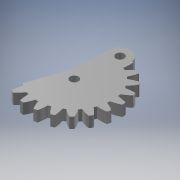
# Autodesk Inventor part: 平歯車2
Saved by Autodesk Inventor 2018 (Build 220112000, 112)
## iProperties
Created: 2017-10-29
Part Number: 平歯車2
Material: Steel
Document SubType Name: Modeling
Designer: sktom
Categories: <?xml version="1.0" encoding="UTF-16"?> <MemberInstance><Categories><FamilyTemplate><FamilyTemplateParameter ValueType="xs:double" Id="1" ObjectReferenceKey="da_z" ObjectType="kUserParameterObject"/><FamilyTemplateParameter ValueType="xs:double" Id="2" ObjectReferenceKey="da_b" ObjectType="kUserParameterObject"/><FamilyTemplateParameter ValueType="xs:double" Id="3" ObjectReferenceKey="da_beta" ObjectType="kUserParameterObject"/><FamilyTemplateParameter ValueType="xs:double" Id="4" ObjectReferenceKey="da_da" ObjectType="kUserParameterObject"/><FamilyTemplateParameter ValueType="xs:double" Id="5" ObjectReferenceKey="da_aw" ObjectType="kUserParameterObject"/><FamilyTemplateParameter ValueType="xs:string" Id="6" ObjectReferenceKey="EAIAABAAAACIAQAAAAAAAIAAAAAAAAAA" ObjectType="83910656" SubObjectId="SurfaceGeometry"/></FamilyTemplate><ParamToTemplateMap><ParamToTemplate CategoryParameter="//CategoryParameter[@InternalName='046C89C9-8512-4d59-83FE-43B91F4F132A']" TemplateParameter="1"/><ParamToTemplate CategoryParameter="//CategoryParameter[@InternalName='2552DF32-E462-4b46-AEBF-C6C7768E72AC']" TemplateParameter="2"/><ParamToTemplate CategoryParameter="//CategoryParameter[@InternalName='C9EE641D-15FC-4fae-A226-E94C4372FDD7']" TemplateParameter="3"/><ParamToTemplate><ParamToTemplate CategoryParameter="//CategoryParameter[@InternalName='00B6519A-459B-49c7-AD84-2E56D39A5744']" ConstantValue="0.000000"/></ParamToTemplate><ParamToTemplate><ParamToTemplate CategoryParameter="//CategoryParameter[@InternalName='04B31F0E-C7A6-4894-AA32-9629BEFACF47']" ConstantValue="1.000000"/></ParamToTemplate><ParamToTemplate><ParamToTemplate CategoryParameter="//CategoryParameter[@InternalName='43CBEC2E-7847-49e7-A936-2F7889FCB2D9']" ConstantValue="0.250000"/></ParamToTemplate><ParamToTemplate><ParamToTemplate CategoryParameter="//CategoryParameter[@InternalName='B1EFC894-105D-4ebd-86BF-FA20ED196853']" ConstantValue="0.350000"/></ParamToTemplate><ParamToTemplate><ParamToTemplate CategoryParameter="//CategoryParameter[@InternalName='51175063-3D10-4879-93E8-6246FE8B403D']" ConstantValue="2060000000.000000"/></ParamToTemplate><ParamToTemplate><ParamToTemplate CategoryParameter="//CategoryParameter[@InternalName='A3A52E27-4454-46a9-B0BD-C932399B70AF']" ConstantValue="0.300000"/></ParamToTemplate><ParamToTemplate><ParamToTemplate CategoryParameter="//CategoryParameter[@InternalName='91B76062-C214-41d9-B1B9-14D2AB99603D']" ConstantValue="0.100000"/></ParamToTemplate><ParamToTemplate><ParamToTemplate CategoryParameter="//CategoryParameter[@InternalName='374E806E-8B8A-4dda-A9AA-1039D6500AD2']" ConstantValue="10.000000"/></ParamToTemplate><ParamToTemplate><ParamToTemplate CategoryParameter="//CategoryParameter[@InternalName='2D373A89-B862-43d6-8D0B-0CBF12AB9F6C']" ConstantValue="0.349066"/></ParamToTemplate><ParamToTemplate CategoryParameter="//CategoryParameter[@InternalName='37777632-D6A2-4fac-9D53-DB8ACD95C989']" TemplateParameter="4"/><ParamToTemplate CategoryParameter="//CategoryParameter[@InternalName='FD1017F1-B727-4f7e-9707-0F86F1FF9423']" TemplateParameter="5"/><ParamToTemplate><ParamToTemplate CategoryParameter="//CategoryParameter[@InternalName='9E1B4470-B2D3-4ff1-B813-535BB4CDF51A']" ConstantValue="3520000.000000"/></ParamToTemplate><ParamToTemplate><ParamToTemplate CategoryParameter="//CategoryParameter[@InternalName='F8452263-BFF6-458c-9FB1-07C4B99E95CD']" ConstantValue="11400000.000000"/></ParamToTemplate><ParamToTemplate><ParamToTemplate CategoryParameter="//CategoryParameter[@InternalName='3E3BB259-FD49-497f-8171-6EBC954A3479']" ConstantValue="2.000000"/></ParamToTemplate><ParamToTemplate CategoryParameter="//CategoryParameter[@InternalName='27C3BAF2-7550-4e4b-AE2C-0DB134B7D9B7']" TemplateParameter="6"/></ParamToTemplateMap><Category DisplayName="Gear" InternalName="DC85795E-93AB-48d5-8EEE-5A27447B64BD" Mnemonic="Gear"><CategoryParameter DisplayName="z" InternalName="046C89C9-8512-4d59-83FE-43B91F4F132A" Mnemonic="z"/><CategoryParameter DisplayName="b" InternalName="2552DF32-E462-4b46-AEBF-C6C7768E72AC" Mnemonic="b"/><CategoryParameter DisplayName="||b|" InternalName="C9EE641D-15FC-4fae-A226-E94C4372FDD7" Mnemonic="beta"/><CategoryParameter DisplayName="x" InternalName="00B6519A-459B-49c7-AD84-2E56D39A5744" Mnemonic="x"/><CategoryParameter DisplayName="a*" InternalName="04B31F0E-C7A6-4894-AA32-9629BEFACF47" Mnemonic="a"/><CategoryParameter DisplayName="c*" InternalName="43CBEC2E-7847-49e7-A936-2F7889FCB2D9" Mnemonic="c"/><CategoryParameter DisplayName="r|.f|*" InternalName="B1EFC894-105D-4ebd-86BF-FA20ED196853" Mnemonic="rf"/><CategoryParameter DisplayName="E" InternalName="51175063-3D10-4879-93E8-6246FE8B403D" Mnemonic="E"/><CategoryParameter DisplayName="||m|" InternalName="A3A52E27-4454-46a9-B0BD-C932399B70AF" Mnemonic="mi"/><Category DisplayName="SpurGear" InternalName="26C5A22E-A91E-4dfd-A3B3-23CCAFAE1764" Mnemonic="SpurGear"><CategoryParameter DisplayName="m" InternalName="91B76062-C214-41d9-B1B9-14D2AB99603D" Mnemonic="m"/><CategoryParameter DisplayName="P" InternalName="374E806E-8B8A-4dda-A9AA-1039D6500AD2" Mnemonic="PP"/><CategoryParameter DisplayName="||a|" InternalName="2D373A89-B862-43d6-8D0B-0CBF12AB9F6C" Mnemonic="alpha"/><CategoryParameter DisplayName="d|.a|" InternalName="37777632-D6A2-4fac-9D53-DB8ACD95C989" Mnemonic="da"/><CategoryParameter DisplayName="a|.w|" InternalName="FD1017F1-B727-4f7e-9707-0F86F1FF9423" Mnemonic="aw"/><CategoryParameter DisplayName="||s||.Flim|" InternalName="9E1B4470-B2D3-4ff1-B813-535BB4CDF51A" Mnemonic="sFlim"/><CategoryParameter DisplayName="||s||.Hlim|" InternalName="F8452263-BFF6-458c-9FB1-07C4B99E95CD" Mnemonic="sHlim"/><CategoryParameter DisplayName="種類" InternalName="3E3BB259-FD49-497f-8171-6EBC954A3479" Mnemonic="type"/><CategoryParameter DisplayName="PitchDiameter" InternalName="27C3BAF2-7550-4e4b-AE2C-0DB134B7D9B7" Mnemonic="IDS_PITCHDIAM"/></Category></Category></Categories></MemberInstance>
Density: 1 g/cm^3
Appearance: Steel
CustomPartVersion: 1
Author: sktom
Autodesk Inventor part; units mm, degrees
ref_plane "YZ Plane" through (0, 0, 0) normal (1, 0, 0) x (0, 1, 0)
ref_plane "XZ Plane" through (0, 0, 0) normal (0, 1, 0) x (-1, 0, 0)
ref_plane "XY Plane" through (0, 0, 0) normal (0, 0, 1) x (1, 0, 0)
sketch "Sketch1" plane through (0, 0, 0) normal (0, 0, 1) x (1, 0, 0)
  circle A0 centre (0, 0) radius 11.5
  dimension "d0" = 23
  constraints: 1 centre point
  measures "d0" diameter of A0
extrude "Extrusion1" add sketch "Sketch1" along normal blind 2.651
ref_plane "Work Plane2" through (0, 0, 1.3255) normal (0, 0, 1) x (1, 0, 0)
sketch "Sketch2" plane through (0, 0, 0) normal (0, 0, -1) x (-1, 0, 0)
  circle A0 centre (0, 0) radius 11.5 projected
  circle A1 centre (0, 0) radius 10.5
  dimension "d3" = 21
  constraints: 1 centre point, 1 coincident
  measures "d3" diameter of A1
surface extrude "ピッチ円直径" sketch "Sketch2" against normal through all shown no curves A1
ref_plane "Work Plane8" through (0, 0, 0) normal (0.9888308, 0.1490423, 0) x (0, 0, 1)
ref_plane "Work Plane9" through (0, 0, 0) normal (1, 0, 0) x (0, 1, 0)
spur gear teeth "平歯車" teeth 21 pitch diameter 21 tip diameter 23 root diameter 18.5 face width 3 start plane through (0, 0, 0) normal (0, 0, -1) x (-1, 0, 0)
sketch "スケッチ3" plane through (0, 0, 2.651) normal (0, 0, 1) x (1, 0, 0)
  circle A0 centre (0, 0) radius 1.05
  dimension "d49" = 2.1
  constraints: 1 centre point, 1 coincident
  measures "d49" diameter of A0
extrude "押し出し2" cut sketch "スケッチ3" against normal through all
sketch "スケッチ4" plane through (0, 0, 2.651) normal (0, 0, 1) x (1, 0, 0)
  circle A0 centre (0.7711, 10.5759) radius 1.05
  circle A1 centre (0.7711, 10.5759) radius 2.651
  line L0 (-1.8729, 10.7687) -> (-2.5842, 1.0131)
  line L1 (-2.5842, 1.0131) -> (-8.2774, -10.3528)
  arc A2 (0.9638, 13.2199) -> (-8.2774, -10.3528) centre (0, 0) ccw
  line L2 (0, 0) -> (-12.3406, 4.8379) construction
  line L3 (0.7711, 10.5759) -> (0, 0) construction
  arc A3 (3.7982, 10.8547) -> (2.9764, 11.1081) centre (0, 0) ccw construction
  point P0 (3.3897, 10.9891)
  dimension "d52" = 10.604
  dimension "d53" = 2.1
  dimension "d54" = 157.563
  dimension "d55" = 2.651
  constraints: 8 end point, 7 point on circle, 3 centre point, 2 coincident, 2 tangent, 1 parallel, 1 point on line
  measures "d52" distance of point (0, 0) A0.centre
  measures "d53" diameter of A0
  measures "d54" angle of L0 L1
  measures "d55" distance from line of point (0, 0) L0
extrude "押し出し3" cut sketch "スケッチ4" against normal through all contours A1 L0 L1 A2
extrude "押し出し4" add sketch "スケッチ4" against normal up to surface (2.651 mm away) contours A1
extrude "押し出し5" cut sketch "スケッチ4" against normal through all contours A0
sketch "スケッチ5" plane through (0, 0, 2.651) normal (0, 0, 1) x (1, 0, 0)
  circle A0 centre (0.7711, 10.5759) radius 2.651 projected
  line L0 (-1.9591, 9.586) -> (-2.5842, 1.0131) projected
  line L1 (-1.8729, 10.7687) -> (-2.5842, 1.0131) projected
  line L2 (0.7711, 10.5759) -> (0, 0) construction
  line L3 (0.5783, 7.9319) -> (-2.0657, 8.1247)
  constraints: 2 end point, 2 point on line, 1 perpendicular, 1 point on circle, 1 tangent
extrude "押し出し6" add sketch "スケッチ5" against normal up to surface (2.651 mm away) contours A0 L3 L0 L1
fillet "フィレット1" radius 0.5 1 edges at (-7.445, -8.6909, 1.3255)
sketch "スケッチ6" plane through (0, 0, 2.651) normal (0, 0, 1) x (1, 0, 0)
  line L0 (-6.6843, -7.1724) -> (-2.5842, 1.0131) projected
  line L1 (-2.5842, 1.0131) -> (-6.9082, -7.6194)
  line L2 (-6.9082, -7.6194) -> (-6.1476, -8.0004)
  arc A0 (-5.4928, -7.4425) -> (-4.9213, -7.8322) centre (0, 0) ccw projected
  line L3 (-6.1476, -8.0004) -> (-5.4928, -7.4425)
  line L4 (-5.4928, -7.4425) -> (-2.5842, 1.0131)
  arc A1 (-6.6843, -7.1724) -> (-5.9392, -7.7978) centre (-6.2373, -7.3963) ccw projected
  arc A2 (-6.6843, -7.1724) -> (-5.9392, -7.7978) centre (-6.2373, -7.3963) ccw construction
  arc A3 (-5.9392, -7.7978) -> (-5.4928, -7.4425) centre (-11.0042, -0.9749) ccw construction
  arc A4 (-5.4928, -7.4425) -> (-4.9213, -7.8322) centre (0, 0) ccw construction
  arc A5 (-4.9213, -7.8322) -> (-5.3736, -10.1673) centre (3.1128, -10.5997) ccw construction
  arc A6 (-5.3736, -10.1673) -> (-4.5988, -10.5405) centre (0, 0) ccw construction
  arc A7 (-4.5988, -10.5405) -> (-3.0551, -8.7309) centre (-10.2279, -4.1751) ccw construction
  arc A8 (-3.0551, -8.7309) -> (-2.3941, -8.9348) centre (0, 0) ccw construction
  arc A9 (-2.3941, -8.9348) -> (-2.138, -11.2995) centre (6.0988, -9.2113) ccw construction
  arc A10 (-2.138, -11.2995) -> (-1.2876, -11.4277) centre (0, 0) ccw construction
  arc A11 (-1.2876, -11.4277) -> (-0.3459, -9.2435) centre (-8.5429, -7.0044) ccw construction
  arc A12 (-0.3459, -9.2435) -> (0.3459, -9.2435) centre (0, 0) ccw construction
  arc A13 (0.3459, -9.2435) -> (1.2876, -11.4277) centre (8.5429, -7.0044) ccw construction
  arc A14 (1.2876, -11.4277) -> (2.138, -11.2995) centre (0, 0) ccw construction
  arc A15 (2.138, -11.2995) -> (2.3941, -8.9348) centre (-6.0988, -9.2113) ccw construction
  arc A16 (2.3941, -8.9348) -> (3.0551, -8.7309) centre (0, 0) ccw construction
  arc A17 (3.0551, -8.7309) -> (4.5988, -10.5405) centre (10.2279, -4.1751) ccw construction
  arc A18 (4.5988, -10.5405) -> (5.3736, -10.1673) centre (0, 0) ccw construction
  arc A19 (5.3736, -10.1673) -> (4.9213, -7.8322) centre (-3.1128, -10.5997) ccw construction
  arc A20 (4.9213, -7.8322) -> (5.4928, -7.4425) centre (0, 0) ccw construction
  arc A21 (5.4928, -7.4425) -> (7.5013, -8.7167) centre (11.0042, -0.9749) ccw construction
  arc A22 (7.5013, -8.7167) -> (8.1317, -8.1317) centre (0, 0) ccw construction
  arc A23 (8.1317, -8.1317) -> (7.0112, -6.0337) centre (0.1498, -11.0463) ccw construction
  arc A24 (7.0112, -6.0337) -> (7.4425, -5.4928) centre (0, 0) ccw construction
  arc A25 (7.4425, -5.4928) -> (9.7373, -6.1184) centre (10.8027, 2.3119) ccw construction
  arc A26 (9.7373, -6.1184) -> (10.1673, -5.3736) centre (0, 0) ccw construction
  arc A27 (10.1673, -5.3736) -> (8.4782, -3.699) centre (3.3991, -10.5114) ccw construction
  arc A28 (8.4782, -3.699) -> (8.7309, -3.0551) centre (0, 0) ccw construction
  arc A29 (8.7309, -3.0551) -> (11.1081, -2.9764) centre (9.6413, 5.3934) ccw construction
  arc A30 (11.1081, -2.9764) -> (11.2995, -2.138) centre (0, 0) ccw construction
  arc A31 (11.2995, -2.138) -> (9.1918, -1.0357) centre (6.3464, -9.0425) ccw construction
  arc A32 (9.1918, -1.0357) -> (9.2435, -0.3459) centre (0, 0) ccw construction
  arc A33 (9.2435, -0.3459) -> (11.492, 0.43) centre (7.6232, 7.9956) ccw construction
  arc A34 (11.492, 0.43) -> (11.4277, 1.2876) centre (0, 0) ccw construction
  arc A35 (11.4277, 1.2876) -> (9.0887, 1.7197) centre (8.7298, -6.7701) ccw construction
  arc A36 (9.0887, 1.7197) -> (8.9348, 2.3941) centre (0, 0) ccw construction
  arc A37 (8.9348, 2.3941) -> (10.8547, 3.7982) centre (4.9278, 9.8873) ccw construction
  arc A38 (10.8547, 3.7982) -> (10.5405, 4.5988) centre (0, 0) ccw construction
  arc A39 (10.5405, 4.5988) -> (8.1781, 4.3222) centre (10.3374, -3.8962) ccw construction
  arc A40 (8.1781, 4.3222) -> (7.8322, 4.9213) centre (0, 0) ccw construction
  arc A41 (7.8322, 4.9213) -> (9.2529, 6.8289) centre (1.7945, 10.9006) ccw construction
  arc A42 (9.2529, 6.8289) -> (8.7167, 7.5013) centre (0, 0) ccw construction
  arc A43 (8.7167, 7.5013) -> (6.5407, 6.5407) centre (11.0266, -0.6761) ccw construction
  arc A44 (6.5407, 6.5407) -> (6.0337, 7.0112) centre (0, 0) ccw construction
  arc A45 (6.0337, 7.0112) -> (6.8289, 9.2529) centre (-1.4982, 10.9452) ccw construction
  arc A46 (6.8289, 9.2529) -> (6.1184, 9.7373) centre (0, 0) ccw construction
  arc A47 (6.1184, 9.7373) -> (4.3222, 8.1781) centre (10.736, 2.6041) ccw construction
  arc A48 (4.3222, 8.1781) -> (3.699, 8.4782) centre (0, 0) ccw construction
  arc A49 (3.699, 8.4782) -> (3.7982, 10.8547) centre (-4.6578, 10.0174) ccw construction
  arc A50 (3.7982, 10.8547) -> (3.3897, 10.9891) centre (0, 0) ccw construction
  arc A51 (3.3897, 10.9891) -> (-1.8729, 10.7687) centre (0.7711, 10.5759) ccw construction
  line L5 (-1.8729, 10.7687) -> (-2.5842, 1.0131) construction
  line L6 (-2.5842, 1.0131) -> (-6.6843, -7.1724) construction
  circle A52 centre (0.7711, 10.5759) radius 1.05 construction
  circle A53 centre (0, 0) radius 1.05 construction
  arc A54 (-5.9392, -7.7978) -> (-5.4928, -7.4425) centre (-11.0042, -0.9749) ccw construction
  constraints: 8 end point, 2 tangent, 1 collinear, 1 perpendicular
extrude "押し出し7" cut sketch "スケッチ6" against normal through all
equation "\"d0\" = da_da"
equation "\"d3\" = da_dw"
equation "\"d16\" = da_aw"
equation "\"d43\" = da_aw"
equation "\"d46\" = da_aw"
equation "\"da_da\" = 23"
equation "\"da_dw\" = 21"
equation "\"da_aw\" = 21.5"
body "Solid1"
body "Srf1"
